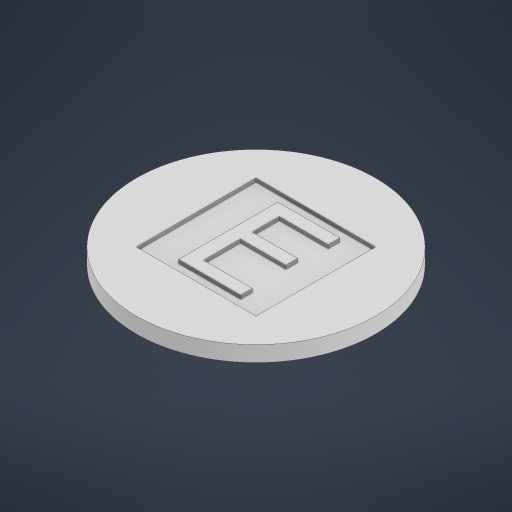
# Autodesk Inventor part: TopMarkerPreset
Saved by Autodesk Inventor 2023.2 (Build 272271030, 271C)
## iProperties
Created: 2023-05-05
Part Number: TopMarkerPreset
Material: Generic
Document SubType Name: Modeling
Designer: Elias Braun
Density: 1 g/cm^3
Appearance: Default
Author: Elias Braun
Autodesk Inventor part; units mm, degrees
ref_plane "YZ Plane" through (0, 0, 0) normal (1, 0, 0) x (0, 1, 0)
ref_plane "XZ Plane" through (0, 0, 0) normal (0, 1, 0) x (-1, 0, 0)
ref_plane "XY Plane" through (0, 0, 0) normal (0, 0, 1) x (1, 0, 0)
sketch "Sketch1" plane through (0, 0, 0) normal (0, 1, 0) x (-1, 0, 0)
  circle A0 centre (0, 0) radius 20
  dimension "d0" = 40
  constraints: 1 centre point, 1 coincident
  measures "d0" diameter of A0
extrude "Extrusion1" add sketch "Sketch1" along normal blind 2.6
sketch "Sketch2" plane through (0, 2.6, 0) normal (0, 1, 0) x (1, 0, 0)
  line L0 (-10, -10) -> (-10, 10)
  line L1 (-10, 10) -> (10, 10)
  line L2 (10, 10) -> (10, -10)
  line L3 (10, -10) -> (-10, -10)
  line L4 (-10, -10) -> (10, 10) construction
  line L5 (-10, 10) -> (10, -10) construction
  point P0 (0, 0)
  dimension "d3" = 20
  dimension "d4" = 20
  constraints: 12 end point, 2 midpoint, 2 parallel, 1 perpendicular, 1 vertical
  measures "d3" distance of L0.start L0.end
  measures "d4" distance of L0.end L1.end
extrude "Extrusion2" cut sketch "Sketch2" against normal blind 0.6
sketch "Sketch3" plane through (0, 2, 0) normal (0, 1, 0) x (1, 0, 0)
  line L0 (-6.3669, 8.3364) -> (6.4396, 8.3364) construction
  line L1 (6.4396, 8.3364) -> (6.4396, -8.2636) construction
  line L2 (6.4396, -8.2636) -> (-6.3669, -8.2636) construction
  line L3 (-6.3669, -8.2636) -> (-6.3669, 8.3364) construction
  line L4 (-4.6854, -8.2636) -> (-4.6854, 8.3364)
  line L5 (-4.6854, 8.3364) -> (5.6997, 8.3364)
  line L6 (5.6997, 8.3364) -> (5.6997, 6.3723)
  line L7 (5.6997, 6.3723) -> (-2.4792, 6.3723)
  line L8 (-2.4792, 6.3723) -> (-2.4792, 1.8255)
  line L9 (-2.4792, 1.8255) -> (5.1482, 1.8255)
  line L10 (5.1482, 1.8255) -> (5.1482, -0.1385)
  line L11 (5.1482, -0.1385) -> (-2.4792, -0.1385)
  line L12 (-2.4792, -0.1385) -> (-2.4792, -6.2996)
  line L13 (-2.4792, -6.2996) -> (5.6997, -6.2996)
  line L14 (5.6997, -6.2996) -> (5.6997, -8.2636)
  line L15 (5.6997, -8.2636) -> (-4.6854, -8.2636)
  point P0 (0, 0)
  constraints: 2 other
extrude "Extrusion3" add sketch "Sketch3" along normal blind 0.6
body "Solid1"
